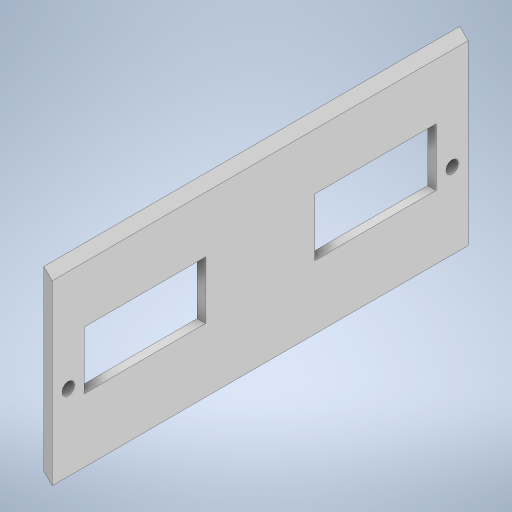
# Autodesk Inventor part: kopia_plug
Saved by Autodesk Inventor 2023 (Build 270158000, 158)
## iProperties
Created: 2023-07-25
Part Number: kopia_plug
Material: Ogólny
Document SubType Name: Modeling
Designer: Kamil
Density: 1 g/cm^3
Appearance: Domyślna
Author: Kamil
Autodesk Inventor part; units mm, degrees
ref_plane "YZ Plane" through (0, 0, 0) normal (1, 0, 0) x (0, 1, 0)
ref_plane "XZ Plane" through (0, 0, 0) normal (0, 1, 0) x (-1, 0, 0)
ref_plane "XY Plane" through (0, 0, 0) normal (0, 0, 1) x (1, 0, 0)
sketch "Szkic1" plane through (0, 0, 0) normal (1, 0, 0) x (0, 1, 0)
  circle A0 centre (18.3256, 3.8503) radius 1.5
  circle A1 centre (18.3256, 96.1497) radius 1.5
  line L0 (15.3555, 36.8868) -> (29.2091, 36.8868)
  line L1 (29.2091, 36.8868) -> (29.2091, 7.7086)
  line L2 (29.2091, 7.7086) -> (15.3555, 7.7086)
  line L3 (15.3555, 7.7086) -> (15.3555, 36.8868)
  line L4 (15.3555, 92.2914) -> (29.2091, 92.2914)
  line L5 (29.2091, 92.2914) -> (29.2091, 63.1132)
  line L6 (29.2091, 63.1132) -> (15.3555, 63.1132)
  line L7 (15.3555, 63.1132) -> (15.3555, 92.2914)
  line L8 (0, 100) -> (43.598, 100)
  line L9 (0, 100) -> (0, 0)
  line L10 (43.598, 0) -> (0, 0)
  line L11 (43.598, 100) -> (43.598, 0)
  line L12 (43.598, 100) -> (44.6676, 100)
  line L13 (43.598, 100) -> (43.598, 0)
  line L14 (44.6676, 0) -> (43.598, 0)
  line L15 (44.6676, 100) -> (44.6676, 0)
  point P0 (33.9001, 100)
  constraints: 32 end point, 2 centre point
extrude "Wyciągnięcie proste1" add sketch "Szkic1" along normal blind 2
chamfer "Faza1" distance 2 angle 45 1 edges at (2, 44.6676, 50)
chamfer "Faza2" distance 2 angle 45 1 edges at (0, 0, 50)
